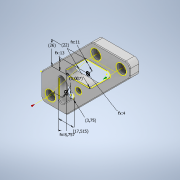
# Autodesk Inventor part: NEW_ACU_FIX2
Saved by Autodesk Inventor 2022 (Build 260153000, 153)
## iProperties
Created: 2021-11-12
Part Number: NEW_ACU_FIX2
Material: Generic
Document SubType Name: Modeling
Designer: Viktor
Density: 1 g/cm^3
Appearance: Default
Author: Viktor
Autodesk Inventor part; units mm, degrees
ref_plane "YZ Plane" through (0, 0, 0) normal (1, 0, 0) x (0, 1, 0)
ref_plane "XZ Plane" through (0, 0, 0) normal (0, 1, 0) x (-1, 0, 0)
ref_plane "XY Plane" through (0, 0, 0) normal (0, 0, 1) x (1, 0, 0)
sketch "Sketch1" plane through (0, 0, 0) normal (0, 0, 1) x (1, 0, 0)
  line L0 (0, 0) -> (0, -56.5685)
  line L1 (0, -56.5685) -> (113.4706, 56.902)
  line L2 (113.4706, 56.902) -> (56.902, 56.902)
  line L3 (56.902, 56.902) -> (0, 0)
  line L4 (-0.4955, 36.902) -> (119.5045, 36.902) construction
  circle A0 centre (89.3284, 46.902) radius 2.25
  circle A1 centre (61.0442, 46.902) radius 2.25
  line L5 (61.0442, 46.902) -> (89.3284, 46.902) construction
  line L6 (20, 35.2608) -> (20, -60.0641) construction
  circle A2 centre (10, -18.2843) radius 2.25
  circle A3 centre (41.5, 1.902) radius 2.75
  dimension "d1" = 40
  dimension "d2" = 20
  dimension "d3" = 10
  dimension "d4" = 4.5
  dimension "d5" = 4.5
  dimension "d6" = 4.5
  dimension "d8" = 5.5
  dimension "d9" = 41.5
  dimension "d10" = 12
  dimension "d11" = 35
  dimension "d12" = 10
  dimension "d14" = 10
  dimension "d17" = 20
  dimension "d18" = 10
  dimension "d19" = 20
  dimension "d20" = 135
  constraints: 14 end point, 4 centre point, 2 horizontal, 2 vertical, 1 parallel, 1 perpendicular
  measures "d1" distance between parallel lines of L1 L3
  measures "d2" distance between parallel lines of L2 L4
  measures "d3" distance between parallel lines of L2 L5
  measures "d4" diameter of A0
  measures "d5" diameter of A1
  measures "d6" diameter of A2
  measures "d8" diameter of A3
  measures "d9" distance from line of L0 A3.centre
  measures "d10" distance from line of L1 A3.centre
  measures "d11" distance from line of L4 A3.centre
  measures "d12" distance from line of L5.end L1
  measures "d14" distance from line of L3 L5.start
  measures "d17" distance between parallel lines of L6 L0
  measures "d18" distance from line of L6 A2.centre
  measures "d19" distance from line of L3 A2.centre
  measures "d20" angle of L0 L1
extrude "Extrusion1" add sketch "Sketch1" along normal blind 10
sketch "Sketch2" plane through (0, 0, 10) normal (0, 0, 1) x (1, 0, 0)
  line L0 (0, -56.5685) -> (113.4706, 56.902) projected
  line L1 (113.4706, 56.902) -> (56.902, 56.902) projected
  line L2 (56.902, 56.902) -> (0, 0) projected
  line L3 (0, 0) -> (0, -56.5685) projected
  circle A0 centre (41.5, 1.902) radius 2.75 projected
  circle A1 centre (10, -18.2843) radius 2.25 projected
  circle A2 centre (61.0442, 46.902) radius 2.25 projected
  circle A3 centre (89.3284, 46.902) radius 2.25 projected
  line L4 (0, -28.2843) -> (28.2843, -28.2843)
  line L5 (99.3284, 56.902) -> (99.3284, 42.7599)
  dimension "d25" = 10
  dimension "d26" = 10
  dimension "d27" = 10
  dimension "d28" = 10
  constraints: 4 end point, 3 point on line, 1 horizontal, 1 midpoint, 1 perpendicular
  measures "d25" distance from line of L3 A1.centre
  measures "d26" distance from line of A1.centre L4
  measures "d27" distance from line of L1 A3.centre
  measures "d28" distance from line of L5 A3.centre
extrude "Extrusion2" cut sketch "Sketch2" against normal through all contours L3 L4 L0 | L5 L1 L0
sketch "Sketch3" plane through (0, 0, 10) normal (0, 0, 1) x (1, 0, 0)
  line L0 (56.902, 56.902) -> (0, 0) projected
  line L1 (99.3284, 56.902) -> (56.902, 56.902) projected
  line L2 (49.6299, 36.902) -> (80.7426, 36.902)
  line L3 (80.7426, 36.902) -> (54.7426, 10.902)
  line L4 (54.7426, 10.902) -> (23.6299, 10.902)
  line L5 (23.6299, 10.902) -> (49.6299, 36.902)
  line L6 (28.2843, -28.2843) -> (99.3284, 42.7599) projected
  circle A0 centre (41.5, 1.902) radius 2.75 projected
  circle A1 centre (61.0442, 46.902) radius 2.25 projected
  dimension "d31" = 9
  dimension "d32" = 9
  dimension "d33" = 20
  dimension "d34" = 9
  dimension "d35" = 10
  constraints: 8 end point, 4 parallel, 1 horizontal
  measures "d31" distance between parallel lines of L0 L5
  measures "d32" distance between parallel lines of L6 L3
  measures "d33" distance between parallel lines of L1 L2
  measures "d34" distance from line of A0.centre L4
  measures "d35" distance from line of A1.centre L2
extrude "Extrusion3" cut sketch "Sketch3" against normal through all contours L2 L3 L4 L5
sketch "Sketch4" plane through (0, 0, 10) normal (0, 0, 1) x (1, 0, 0)
  line L0 (20, 1) -> (20, -23.8406)
  line L1 (20, -23.8406) -> (37.2574, -6.5833)
  line L2 (37.2574, -6.5833) -> (21.701, 8.9731)
  line L3 (0, 0) -> (0, -28.2843) projected
  line L4 (28.2843, -28.2843) -> (99.3284, 42.7599) projected
  line L5 (80.7426, 36.902) -> (54.7426, 10.902) projected
  line L6 (56.902, 56.902) -> (0, 0) projected
  line L7 (21.701, 8.9731) -> (20, 7.2721)
  line L8 (20, 7.2721) -> (20, 1)
  circle A0 centre (41.5, 1.902) radius 2.75 projected
  dimension "d39" = 20
  dimension "d41" = 9
  dimension "d42" = 9
  dimension "d43" = 9
  dimension "d44" = 90
  dimension "d45" = 9
  dimension "d46" = 90
  constraints: 10 end point, 1 collinear, 1 parallel, 1 vertical
  measures "d39" distance between parallel lines of L3 L0
  measures "d41" distance between parallel lines of L4 L1
  measures "d42" distance between parallel lines of L4 L5
  measures "d43" distance from line of L6 L2.end
  measures "d44" angle of L2 L1
  measures "d45" distance from line of A0.centre L2
  measures "d46" angle of L2 L7
extrude "Extrusion4" cut sketch "Sketch4" against normal through all contours L8 L7 L2 L1 L0
sketch "Sketch5" plane through (0, 0, 10) normal (0, 0, 1) x (1, 0, 0)
  circle A0 centre (10, -18.2843) radius 2.25 projected
  circle A1 centre (41.5, 1.902) radius 2.75 projected
  circle A2 centre (61.0442, 46.902) radius 2.25 projected
  circle A3 centre (89.3284, 46.902) radius 2.25 projected
  circle A4 centre (10, -18.2843) radius 5
  circle A5 centre (61.0442, 46.902) radius 5
  circle A6 centre (89.3284, 46.902) radius 5
  point P0 (0, 0)
  dimension "d49" = 10
  dimension "d50" = 10
  dimension "d51" = 10
  constraints: 3 centre point, 3 coincident
  measures "d49" diameter of A5
  measures "d50" diameter of A6
  measures "d51" diameter of A4
extrude "Extrusion5" cut sketch "Sketch5" against normal blind 5.5 contours A2 | A4 | A5 | A6
sketch "Sketch6" plane through (0, 0, 0) normal (0, 0, -1) x (-1, 0, 0)
  circle A0 centre (-41.5, 1.902) radius 2.75 projected
  line L0 (-44.9293, -1.5273) -> (-46.1845, 3.1572)
  line L1 (-46.1845, 3.1572) -> (-42.7552, 6.5865)
  line L2 (-42.7552, 6.5865) -> (-38.0707, 5.3313)
  line L3 (-38.0707, 5.3313) -> (-36.8155, 0.6468)
  line L4 (-36.8155, 0.6468) -> (-40.2448, -2.7825)
  line L5 (-40.2448, -2.7825) -> (-44.9293, -1.5273)
  line L6 (-37.2574, -6.5833) -> (-21.701, 8.9731) projected
  point P0 (0, 0)
  dimension "d54" = 8.4
  constraints: 12 end point, 1 coincident, 1 parallel, 13 other
  measures "d54" distance between parallel lines of L2 L5
extrude "Extrusion6" cut sketch "Sketch6" against normal blind 3.8
sketch "Sketch7" plane through (0, 0, 0) normal (0, 0, -1) x (-1, 0, 0)
  line L0 (-42.7552, 6.5865) -> (-38.0707, 5.3313) projected
  line L1 (-40.2448, -2.7825) -> (-44.9293, -1.5273) projected
  line L2 (-42.7552, 6.5865) -> (-40.2448, -2.7825) construction
  circle A0 centre (-40.5683, -1.5751) radius 1.25
  point P0 (0, 0)
  dimension "d57" = 2.5
  constraints: 2 end point, 1 point on line, 3 other
extrude "Extrusion7" cut sketch "Sketch7" against normal up to surface (3.8 mm away)
pattern_circular "Circular Pattern1" count 6 over 360 about axis through (41.5, 1.902, 0) along (0, 0, 1) of "Extrusion7"
fillet "Fillet1" radius 3 8 edges at (21.701, 8.9731, 5) (20, 7.2721, 5) (20, -23.8406, 5) (37.2574, -6.5833, 5) (54.7426, 10.902, 5) (80.7426, 36.902, 5) (49.6299, 36.902, 5) (23.6299, 10.902, 5)
fillet "Fillet2" radius 5 6 edges at (99.3284, 42.7599, 5) (99.3284, 56.902, 5) (56.902, 56.902, 5) (0, 0, 5) (0, -28.2843, 5) (28.2843, -28.2843, 5)
chamfer "Chamfer1" distance 0.75 angle 45 30 edges at (28.451, 28.451, 10) (0.3806, -0.1577, 10) (0, -12.6777, 10) (1.4645, -26.8198, 10) (15.6066, -28.2843, 10) (28.1266, -27.9037, 10) (63.8063, 7.2378, 10) (98.9478, 42.9175, 10) (99.3284, 48.3665, 10) (97.864, 55.4376, 10) (76.6508, 56.902, 10) (57.0597, 56.5214, 10) (5, -18.2843, 10) (30.1287, 0.5454, 10) (36.0147, -6.5833, 10) (30.1287, -13.7119, 10) (21.8519, -19.3696, 10) (20, -6.5833, 10) (21.8519, 6.2031, 10) (38.75, 1.902, 10) (62.1863, 36.902, 10) (76.2716, 35.0501, 10) (65.6213, 21.7807, 10) (54.6481, 11.1304, 10) (42.1863, 10.902, 10) (28.1009, 12.754, 10) (38.7513, 26.0233, 10) (49.7245, 36.6737, 10) (56.0442, 46.902, 10) (84.3284, 46.902, 10)
sketch "Sketch8" plane through (0, 0, 10) normal (0, 0, 1) x (1, 0, 0)
  circle A0 centre (61.0442, 46.902) radius 5.75 projected
  circle A1 centre (89.3284, 46.902) radius 5.75 projected
  circle A2 centre (10, -18.2843) radius 5.75 projected
  circle A3 centre (41.5, 1.902) radius 3.5 projected
  arc A4 (76.1517, 31.2504) -> (73.5, 37.652) centre (73.5, 33.902) ccw projected
  arc A5 (35.6664, -9.2349) -> (35.6664, -3.9316) centre (33.0147, -6.5833) ccw projected
  point P0 (0, 0)
sketch "Sketch9" plane through (0, 0, 10) normal (0, 0, 1) x (1, 0, 0)
  circle A0 centre (52.1863, 23.902) radius 2
  circle A1 centre (28.0074, -6.5833) radius 2
  line L0 (20, -16.598) -> (20, 3.4315) projected
  arc A2 (35.6664, -9.2349) -> (35.6664, -3.9316) centre (33.0147, -6.5833) ccw projected
  line L1 (19.25, 3.4315) -> (19.25, -16.598) projected
  line L2 (28.7513, 16.0233) -> (48.7513, 36.0233) projected
  line L3 (75.6213, 31.7807) -> (55.6213, 11.7807) projected
  line L4 (50.8726, 36.902) -> (73.5, 36.902) projected
  line L5 (53.5, 10.902) -> (30.8726, 10.902) projected
  point P0 (0, 0)
  dimension "d70" = 0
  dimension "d71" = 5.0074
  dimension "d72" = 8.7574
  dimension "d73" = 17.5147
  dimension "d74" = 3.75
  dimension "d75" = 4
  dimension "d76" = 11
  dimension "d77" = 22
  dimension "d78" = 26
  dimension "d79" = 13
  dimension "d80" = 4
  constraints: 2 centre point
  measures "d70" vertical distance of A2.centre A1.centre
  measures "d71" distance of A2.centre A1.centre
  measures "d72" distance from line of A1.centre L1
  measures "d74" radius of A2
  measures "d75" diameter of A1
  measures "d76" distance from line of L2 A0.centre
  measures "d77" distance between parallel lines of L2 L3
  measures "d78" distance between parallel lines of L4 L5
  measures "d79" distance from line of L5 A0.centre
  measures "d80" diameter of A0
equation "\"d4\" = d5"
equation "\"d6\" = d5"
equation "\"d12\" = d14"
equation "\"d19\" = 0.5 * d1"
equation "\"d26\" = d25"
equation "\"d28\" = d27"
equation "\"d32\" = d31"
equation "\"d34\" = d31"
equation "\"d41\" = d42"
equation "\"d43\" = d41"
equation "\"d45\" = d41"
equation "\"d51\" = d49"
equation "\"d72\" = 0.5 * d73"
equation "\"d76\" = 0.5 * d77"
equation "\"d79\" = 0.5 * d78"
equation "\"d80\" = d75"
body "Solid1"
